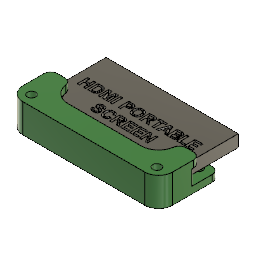
screen_holder (Autodesk Fusion 360 design; units mm, degrees)
Autodesk Fusion 360 part; units mm, degrees
sketch "Sketch1" plane through (0, 0, 0) normal (0, 0, 1) x (1, 0, 0) in component "screen"
  line L0 (95, 57.5) -> (-95, 57.5)
  line L1 (-95, 57.5) -> (-95, -57.5)
  line L2 (-95, -57.5) -> (95, -57.5)
  line L3 (95, -57.5) -> (95, 57.5)
  line L4 (95, 57.5) -> (-95, -57.5) construction
  line L5 (-95, 57.5) -> (95, -57.5) construction
  dimension "d1" = 190
  dimension "d2" = 115
  constraint horizontal L0
  constraint perpendicular L0 L1
  constraint parallel L0 L2
  constraint parallel L1 L3
  constraint coincident L4 origin
  constraint coincident L5 origin
  measures "d1" distance of L1.end L2.end
  measures "d2" distance of L0.end L1.end
extrude "Extrude1" add sketch "Sketch1" along normal blind 17.5 makes body 1 in component "screen"
sketch "Sketch2" plane through (0, 0, 17.5) normal (0, 0, 1) x (-1, 0, 0) in component "screen"
  line L0 (-95, 57.5) -> (-95, -57.5)
  line L1 (-95, -57.5) -> (95, -57.5)
  line L2 (95, -57.5) -> (95, 57.5)
  line L3 (95, 57.5) -> (-95, 57.5)
  line L4 (82.8095, -4.1103) -> (82.8095, -18.9885)
  line L5 (82.8095, -18.9885) -> (79.8055, -18.9885)
  line L6 (79.8055, -18.9885) -> (79.8055, -13.1326)
  line L7 (79.8055, -13.1326) -> (73.9191, -13.1326)
  line L8 (73.9191, -13.1326) -> (73.9191, -18.9885)
  line L9 (73.9191, -18.9885) -> (70.9151, -18.9885)
  line L10 (70.9151, -18.9885) -> (70.9151, -4.1103)
  line L11 (70.9151, -4.1103) -> (73.9191, -4.1103)
  line L12 (73.9191, -4.1103) -> (73.9191, -10.6157)
  line L13 (73.9191, -10.6157) -> (79.8055, -10.6157)
  line L14 (79.8055, -10.6157) -> (79.8055, -4.1103)
  line L15 (79.8055, -4.1103) -> (82.8095, -4.1103)
  line L16 (67.8095, -18.9885) -> (62.319, -18.9885)
  spline S0 degree 2 poles (62.319, -18.9885) (60.4618, -18.9885) (59.4875, -18.7043) knots 0 0 0 1 1 1
  spline S1 degree 2 poles (59.4875, -18.7043) (58.1783, -18.3187) (57.2446, -17.3342) knots 0 0 0 1 1 1
  spline S2 degree 2 poles (57.2446, -17.3342) (56.3109, -16.3498) (55.8237, -14.9239) knots 0 0 0 1 1 1
  spline S3 degree 2 poles (55.8237, -14.9239) (55.3366, -13.498) (55.3366, -11.4073) knots 0 0 0 1 1 1
  spline S4 degree 2 poles (55.3366, -11.4073) (55.3366, -9.5704) (55.7933, -8.2409) knots 0 0 0 1 1 1
  spline S5 degree 2 poles (55.7933, -8.2409) (56.3515, -6.617) (57.3867, -5.6123) knots 0 0 0 1 1 1
  spline S6 degree 2 poles (57.3867, -5.6123) (58.1681, -4.8511) (59.4976, -4.4249) knots 0 0 0 1 1 1
  spline S7 degree 2 poles (59.4976, -4.4249) (60.4922, -4.1103) (62.1566, -4.1103) knots 0 0 0 1 1 1
  line L17 (62.1566, -4.1103) -> (67.8095, -4.1103)
  line L18 (67.8095, -4.1103) -> (67.8095, -18.9885)
  line L19 (64.8055, -16.4716) -> (64.8055, -6.617)
  line L20 (64.8055, -6.617) -> (62.5626, -6.617)
  spline S8 degree 2 poles (62.5626, -6.617) (61.3041, -6.617) (60.7459, -6.7591) knots 0 0 0 1 1 1
  spline S9 degree 2 poles (60.7459, -6.7591) (60.0152, -6.9418) (59.5331, -7.3782) knots 0 0 0 1 1 1
  spline S10 degree 2 poles (59.5331, -7.3782) (59.0511, -7.8146) (58.7466, -8.8143) knots 0 0 0 1 1 1
  spline S11 degree 2 poles (58.7466, -8.8143) (58.4421, -9.8139) (58.4421, -11.5392) knots 0 0 0 1 1 1
  spline S12 degree 2 poles (58.4421, -11.5392) (58.4421, -13.2645) (58.7466, -14.1881) knots 0 0 0 1 1 1
  spline S13 degree 2 poles (58.7466, -14.1881) (59.0511, -15.1116) (59.5991, -15.6292) knots 0 0 0 1 1 1
  spline S14 degree 2 poles (59.5991, -15.6292) (60.1471, -16.1468) (60.9895, -16.3295) knots 0 0 0 1 1 1
  spline S15 degree 2 poles (60.9895, -16.3295) (61.6187, -16.4716) (63.4557, -16.4716) knots 0 0 0 1 1 1
  line L21 (63.4557, -16.4716) -> (64.8055, -16.4716)
  line L22 (52.8197, -4.1103) -> (52.8197, -18.9885)
  line L23 (52.8197, -18.9885) -> (48.3237, -18.9885)
  line L24 (48.3237, -18.9885) -> (45.6241, -8.8396)
  line L25 (45.6241, -8.8396) -> (42.955, -18.9885)
  line L26 (42.955, -18.9885) -> (38.4489, -18.9885)
  line L27 (38.4489, -18.9885) -> (38.4489, -4.1103)
  line L28 (38.4489, -4.1103) -> (41.2398, -4.1103)
  line L29 (41.2398, -4.1103) -> (41.2398, -15.822)
  line L30 (41.2398, -15.822) -> (44.1932, -4.1103)
  line L31 (44.1932, -4.1103) -> (47.0856, -4.1103)
  line L32 (47.0856, -4.1103) -> (50.0287, -15.822)
  line L33 (50.0287, -15.822) -> (50.0287, -4.1103)
  line L34 (50.0287, -4.1103) -> (52.8197, -4.1103)
  line L35 (35.5463, -4.1103) -> (35.5463, -18.9885)
  line L36 (35.5463, -18.9885) -> (32.5423, -18.9885)
  line L37 (32.5423, -18.9885) -> (32.5423, -4.1103)
  line L38 (32.5423, -4.1103) -> (35.5463, -4.1103)
  line L39 (23.8853, -4.1103) -> (23.8853, -18.9885)
  line L40 (23.8853, -18.9885) -> (19.0646, -18.9885)
  spline S16 degree 2 poles (19.0646, -18.9885) (16.3244, -18.9885) (15.4922, -18.7652) knots 0 0 0 1 1 1
  spline S17 degree 2 poles (15.4922, -18.7652) (14.2134, -18.4303) (13.3508, -17.3089) knots 0 0 0 1 1 1
  spline S18 degree 2 poles (13.3508, -17.3089) (12.4882, -16.1874) (12.4882, -14.4114) knots 0 0 0 1 1 1
  spline S19 degree 2 poles (12.4882, -14.4114) (12.4882, -13.0413) (12.9854, -12.1076) knots 0 0 0 1 1 1
  spline S20 degree 2 poles (12.9854, -12.1076) (13.4827, -11.1739) (14.249, -10.6411) knots 0 0 0 1 1 1
  spline S21 degree 2 poles (14.249, -10.6411) (15.0152, -10.1083) (15.8068, -9.9357) knots 0 0 0 1 1 1
  spline S22 degree 2 poles (15.8068, -9.9357) (16.8826, -9.7226) (18.9225, -9.7226) knots 0 0 0 1 1 1
  line L41 (18.9225, -9.7226) -> (20.8812, -9.7226)
  line L42 (20.8812, -9.7226) -> (20.8812, -4.1103)
  line L43 (20.8812, -4.1103) -> (23.8853, -4.1103)
  line L44 (20.8812, -16.4716) -> (20.8812, -12.2497)
  line L45 (20.8812, -12.2497) -> (19.2371, -12.2497)
  spline S23 degree 2 poles (19.2371, -12.2497) (17.4611, -12.2497) (16.8623, -12.4831) knots 0 0 0 1 1 1
  spline S24 degree 2 poles (16.8623, -12.4831) (16.2635, -12.7165) (15.9235, -13.2138) knots 0 0 0 1 1 1
  spline S25 degree 2 poles (15.9235, -13.2138) (15.5836, -13.7111) (15.5836, -14.3708) knots 0 0 0 1 1 1
  spline S26 degree 2 poles (15.5836, -14.3708) (15.5836, -15.1827) (16.0605, -15.7104) knots 0 0 0 1 1 1
  spline S27 degree 2 poles (16.0605, -15.7104) (16.5375, -16.2382) (17.2683, -16.3701) knots 0 0 0 1 1 1
  spline S28 degree 2 poles (17.2683, -16.3701) (17.8061, -16.4716) (19.43, -16.4716) knots 0 0 0 1 1 1
  line L46 (19.43, -16.4716) -> (20.8812, -16.4716)
  spline S29 degree 2 poles (10.6208, -11.458) (10.6208, -13.7314) (9.9408, -15.274) knots 0 0 0 1 1 1
  spline S30 degree 2 poles (9.9408, -15.274) (9.4333, -16.4107) (8.5555, -17.3139) knots 0 0 0 1 1 1
  spline S31 degree 2 poles (8.5555, -17.3139) (7.6776, -18.2172) (6.6323, -18.6536) knots 0 0 0 1 1 1
  spline S32 degree 2 poles (6.6323, -18.6536) (5.2419, -19.2422) (3.4252, -19.2422) knots 0 0 0 1 1 1
  spline S33 degree 2 poles (3.4252, -19.2422) (0.137, -19.2422) (-1.837, -17.2023) knots 0 0 0 1 1 1
  spline S34 degree 2 poles (-1.837, -17.2023) (-3.8109, -15.1624) (-3.8109, -11.5291) knots 0 0 0 1 1 1
  spline S35 degree 2 poles (-3.8109, -11.5291) (-3.8109, -7.9262) (-1.8522, -5.8914) knots 0 0 0 1 1 1
  spline S36 degree 2 poles (-1.8522, -5.8914) (0.1066, -3.8566) (3.3846, -3.8566) knots 0 0 0 1 1 1
  spline S37 degree 2 poles (3.3846, -3.8566) (6.7033, -3.8566) (8.662, -5.8813) knots 0 0 0 1 1 1
  spline S38 degree 2 poles (8.662, -5.8813) (10.6208, -7.906) (10.6208, -11.458) knots 0 0 0 1 1 1
  spline S39 degree 2 poles (7.5254, -11.5595) (7.5254, -9.0325) (6.3582, -7.7283) knots 0 0 0 1 1 1
  spline S40 degree 2 poles (6.3582, -7.7283) (5.1911, -6.4242) (3.3948, -6.4242) knots 0 0 0 1 1 1
  spline S41 degree 2 poles (3.3948, -6.4242) (1.5984, -6.4242) (0.4465, -7.7182) knots 0 0 0 1 1 1
  spline S42 degree 2 poles (0.4465, -7.7182) (-0.7053, -9.0122) (-0.7053, -11.6001) knots 0 0 0 1 1 1
  spline S43 degree 2 poles (-0.7053, -11.6001) (-0.7053, -14.1576) (0.4161, -15.4161) knots 0 0 0 1 1 1
  spline S44 degree 2 poles (0.4161, -15.4161) (1.5375, -16.6746) (3.3948, -16.6746) knots 0 0 0 1 1 1
  spline S45 degree 2 poles (3.3948, -16.6746) (5.252, -16.6746) (6.3887, -15.4009) knots 0 0 0 1 1 1
  spline S46 degree 2 poles (6.3887, -15.4009) (7.5254, -14.1272) (7.5254, -11.5595) knots 0 0 0 1 1 1
  line L47 (-6.1756, -4.1103) -> (-6.1756, -18.9885)
  line L48 (-6.1756, -18.9885) -> (-12.4983, -18.9885)
  spline S47 degree 2 poles (-12.4983, -18.9885) (-14.8833, -18.9885) (-15.9641, -18.5876) knots 0 0 0 1 1 1
  spline S48 degree 2 poles (-15.9641, -18.5876) (-17.045, -18.1867) (-17.6945, -17.1617) knots 0 0 0 1 1 1
  spline S49 degree 2 poles (-17.6945, -17.1617) (-18.3441, -16.1367) (-18.3441, -14.8173) knots 0 0 0 1 1 1
  spline S50 degree 2 poles (-18.3441, -14.8173) (-18.3441, -13.1428) (-17.3596, -12.0518) knots 0 0 0 1 1 1
  spline S51 degree 2 poles (-17.3596, -12.0518) (-16.3752, -10.9608) (-14.4164, -10.6766) knots 0 0 0 1 1 1
  spline S52 degree 2 poles (-14.4164, -10.6766) (-15.3907, -10.1083) (-16.025, -9.4283) knots 0 0 0 1 1 1
  spline S53 degree 2 poles (-16.025, -9.4283) (-16.6593, -8.7483) (-17.7351, -7.0128) knots 0 0 0 1 1 1
  line L49 (-17.7351, -7.0128) -> (-19.5518, -4.1103)
  line L50 (-19.5518, -4.1103) -> (-15.9591, -4.1103)
  line L51 (-15.9591, -4.1103) -> (-13.7872, -7.3478)
  spline S54 degree 2 poles (-13.7872, -7.3478) (-12.6303, -9.0832) (-12.204, -9.5348) knots 0 0 0 1 1 1
  spline S55 degree 2 poles (-12.204, -9.5348) (-11.7778, -9.9865) (-11.3008, -10.1539) knots 0 0 0 1 1 1
  spline S56 degree 2 poles (-11.3008, -10.1539) (-10.8238, -10.3214) (-9.7886, -10.3214) knots 0 0 0 1 1 1
  line L52 (-9.7886, -10.3214) -> (-9.1796, -10.3214)
  line L53 (-9.1796, -10.3214) -> (-9.1796, -4.1103)
  line L54 (-9.1796, -4.1103) -> (-6.1756, -4.1103)
  line L55 (-9.1796, -12.6962) -> (-11.4022, -12.6962)
  spline S57 degree 2 poles (-11.4022, -12.6962) (-13.5639, -12.6962) (-14.1018, -12.8789) knots 0 0 0 1 1 1
  spline S58 degree 2 poles (-14.1018, -12.8789) (-14.6397, -13.0616) (-14.9442, -13.5081) knots 0 0 0 1 1 1
  spline S59 degree 2 poles (-14.9442, -13.5081) (-15.2487, -13.9547) (-15.2487, -14.6245) knots 0 0 0 1 1 1
  spline S60 degree 2 poles (-15.2487, -14.6245) (-15.2487, -15.3755) (-14.8478, -15.8373) knots 0 0 0 1 1 1
  spline S61 degree 2 poles (-14.8478, -15.8373) (-14.4469, -16.299) (-13.7162, -16.4208) knots 0 0 0 1 1 1
  spline S62 degree 2 poles (-13.7162, -16.4208) (-13.3508, -16.4716) (-11.524, -16.4716) knots 0 0 0 1 1 1
  line L56 (-11.524, -16.4716) -> (-9.1796, -16.4716)
  line L57 (-9.1796, -16.4716) -> (-9.1796, -12.6962)
  line L58 (-24.1593, -4.1103) -> (-24.1593, -16.4716)
  line L59 (-24.1593, -16.4716) -> (-19.7446, -16.4716)
  line L60 (-19.7446, -16.4716) -> (-19.7446, -18.9885)
  line L61 (-19.7446, -18.9885) -> (-31.568, -18.9885)
  line L62 (-31.568, -18.9885) -> (-31.568, -16.4716)
  line L63 (-31.568, -16.4716) -> (-27.1634, -16.4716)
  line L64 (-27.1634, -16.4716) -> (-27.1634, -4.1103)
  line L65 (-27.1634, -4.1103) -> (-24.1593, -4.1103)
  line L66 (-45.3907, -4.1103) -> (-42.1228, -4.1103)
  line L67 (-42.1228, -4.1103) -> (-40.8238, -7.4898)
  line L68 (-40.8238, -7.4898) -> (-34.8765, -7.4898)
  line L69 (-34.8765, -7.4898) -> (-33.6485, -4.1103)
  line L70 (-33.6485, -4.1103) -> (-30.4618, -4.1103)
  line L71 (-30.4618, -4.1103) -> (-36.2568, -18.9885)
  line L72 (-36.2568, -18.9885) -> (-39.4334, -18.9885)
  line L73 (-39.4334, -18.9885) -> (-45.3907, -4.1103)
  line L74 (-39.8596, -9.9966) -> (-37.8095, -15.5176)
  line L75 (-37.8095, -15.5176) -> (-35.8001, -9.9966)
  line L76 (-35.8001, -9.9966) -> (-39.8596, -9.9966)
  line L77 (-45.8576, -18.9885) -> (-51.8048, -18.9885)
  spline S63 degree 2 poles (-51.8048, -18.9885) (-53.5707, -18.9885) (-54.4384, -18.8413) knots 0 0 0 1 1 1
  spline S64 degree 2 poles (-54.4384, -18.8413) (-55.3062, -18.6942) (-55.9912, -18.2273) knots 0 0 0 1 1 1
  spline S65 degree 2 poles (-55.9912, -18.2273) (-56.6763, -17.7605) (-57.133, -16.9841) knots 0 0 0 1 1 1
  spline S66 degree 2 poles (-57.133, -16.9841) (-57.5897, -16.2077) (-57.5897, -15.2436) knots 0 0 0 1 1 1
  spline S67 degree 2 poles (-57.5897, -15.2436) (-57.5897, -14.1982) (-57.0264, -13.3254) knots 0 0 0 1 1 1
  spline S68 degree 2 poles (-57.0264, -13.3254) (-56.4631, -12.4526) (-55.499, -12.0162) knots 0 0 0 1 1 1
  spline S69 degree 2 poles (-55.499, -12.0162) (-56.8589, -11.6204) (-57.5897, -10.6664) knots 0 0 0 1 1 1
  spline S70 degree 2 poles (-57.5897, -10.6664) (-58.3204, -9.7124) (-58.3204, -8.4235) knots 0 0 0 1 1 1
  spline S71 degree 2 poles (-58.3204, -8.4235) (-58.3204, -7.4087) (-57.8484, -6.4496) knots 0 0 0 1 1 1
  spline S72 degree 2 poles (-57.8484, -6.4496) (-57.3765, -5.4905) (-56.5595, -4.9171) knots 0 0 0 1 1 1
  spline S73 degree 2 poles (-56.5595, -4.9171) (-55.7426, -4.3437) (-54.545, -4.2118) knots 0 0 0 1 1 1
  spline S74 degree 2 poles (-54.545, -4.2118) (-53.794, -4.1306) (-50.9219, -4.1103) knots 0 0 0 1 1 1
  line L78 (-50.9219, -4.1103) -> (-45.8576, -4.1103)
  line L79 (-45.8576, -4.1103) -> (-45.8576, -18.9885)
  line L80 (-48.8616, -16.5122) -> (-48.8616, -13.0717)
  line L81 (-48.8616, -13.0717) -> (-50.8305, -13.0717)
  spline S75 degree 2 poles (-50.8305, -13.0717) (-52.5863, -13.0717) (-53.0125, -13.1225) knots 0 0 0 1 1 1
  spline S76 degree 2 poles (-53.0125, -13.1225) (-53.7838, -13.2138) (-54.2253, -13.6553) knots 0 0 0 1 1 1
  spline S77 degree 2 poles (-54.2253, -13.6553) (-54.6668, -14.0967) (-54.6668, -14.8173) knots 0 0 0 1 1 1
  spline S78 degree 2 poles (-54.6668, -14.8173) (-54.6668, -15.5074) (-54.2862, -15.9388) knots 0 0 0 1 1 1
  spline S79 degree 2 poles (-54.2862, -15.9388) (-53.9056, -16.3701) (-53.1546, -16.4614) knots 0 0 0 1 1 1
  spline S80 degree 2 poles (-53.1546, -16.4614) (-52.7081, -16.5122) (-50.587, -16.5122) knots 0 0 0 1 1 1
  line L82 (-50.587, -16.5122) -> (-48.8616, -16.5122)
  line L83 (-48.8616, -10.5954) -> (-48.8616, -6.617)
  line L84 (-48.8616, -6.617) -> (-51.6424, -6.617)
  spline S81 degree 2 poles (-51.6424, -6.617) (-53.2662, -6.617) (-53.7026, -6.7084) knots 0 0 0 1 1 1
  spline S82 degree 2 poles (-53.7026, -6.7084) (-54.3725, -6.8302) (-54.7936, -7.3021) knots 0 0 0 1 1 1
  spline S83 degree 2 poles (-54.7936, -7.3021) (-55.2148, -7.774) (-55.2148, -8.5656) knots 0 0 0 1 1 1
  spline S84 degree 2 poles (-55.2148, -8.5656) (-55.2148, -9.2354) (-54.8901, -9.7023) knots 0 0 0 1 1 1
  spline S85 degree 2 poles (-54.8901, -9.7023) (-54.5653, -10.1691) (-53.9513, -10.3823) knots 0 0 0 1 1 1
  spline S86 degree 2 poles (-53.9513, -10.3823) (-53.3373, -10.5954) (-51.2872, -10.5954) knots 0 0 0 1 1 1
  line L85 (-51.2872, -10.5954) -> (-48.8616, -10.5954)
  line L86 (-59.8021, -4.1103) -> (-59.8021, -18.8667)
  line L87 (-59.8021, -18.8667) -> (-62.8062, -18.8667)
  line L88 (-62.8062, -18.8667) -> (-62.8062, -6.617)
  line L89 (-62.8062, -6.617) -> (-70.2757, -6.617)
  line L90 (-70.2757, -6.617) -> (-70.2757, -4.1103)
  line L91 (-70.2757, -4.1103) -> (-59.8021, -4.1103)
  line L92 (-71.2906, -4.1103) -> (-71.2906, -18.9885)
  line L93 (-71.2906, -18.9885) -> (-82.3224, -18.9885)
  line L94 (-82.3224, -18.9885) -> (-82.3224, -16.4716)
  line L95 (-82.3224, -16.4716) -> (-74.2946, -16.4716)
  line L96 (-74.2946, -16.4716) -> (-74.2946, -13.1732)
  line L97 (-74.2946, -13.1732) -> (-81.7642, -13.1732)
  line L98 (-81.7642, -13.1732) -> (-81.7642, -10.6664)
  line L99 (-81.7642, -10.6664) -> (-74.2946, -10.6664)
  line L100 (-74.2946, -10.6664) -> (-74.2946, -6.617)
  line L101 (-74.2946, -6.617) -> (-82.6066, -6.617)
  line L102 (-82.6066, -6.617) -> (-82.6066, -4.1103)
  line L103 (-82.6066, -4.1103) -> (-71.2906, -4.1103)
  line L104 (42.9296, 14.2693) -> (40.0068, 13.9851)
  spline S87 degree 2 poles (40.0068, 13.9851) (39.7429, 15.4567) (38.9361, 16.1468) knots 0 0 0 1 1 1
  spline S88 degree 2 poles (38.9361, 16.1468) (38.1292, 16.8369) (36.7591, 16.8369) knots 0 0 0 1 1 1
  spline S89 degree 2 poles (36.7591, 16.8369) (35.3078, 16.8369) (34.5721, 16.2229) knots 0 0 0 1 1 1
  spline S90 degree 2 poles (34.5721, 16.2229) (33.8363, 15.6089) (33.8363, 14.7869) knots 0 0 0 1 1 1
  spline S91 degree 2 poles (33.8363, 14.7869) (33.8363, 14.2591) (34.1458, 13.8887) knots 0 0 0 1 1 1
  spline S92 degree 2 poles (34.1458, 13.8887) (34.4553, 13.5183) (35.2266, 13.2443) knots 0 0 0 1 1 1
  spline S93 degree 2 poles (35.2266, 13.2443) (35.7544, 13.0616) (37.6319, 12.5947) knots 0 0 0 1 1 1
  spline S94 degree 2 poles (37.6319, 12.5947) (40.0474, 11.9959) (41.0216, 11.1231) knots 0 0 0 1 1 1
  spline S95 degree 2 poles (41.0216, 11.1231) (42.3917, 9.8951) (42.3917, 8.1292) knots 0 0 0 1 1 1
  spline S96 degree 2 poles (42.3917, 8.1292) (42.3917, 6.9926) (41.7473, 6.0031) knots 0 0 0 1 1 1
  spline S97 degree 2 poles (41.7473, 6.0031) (41.1028, 5.0135) (39.89, 4.4959) knots 0 0 0 1 1 1
  spline S98 degree 2 poles (39.89, 4.4959) (38.6773, 3.9784) (36.9621, 3.9784) knots 0 0 0 1 1 1
  spline S99 degree 2 poles (36.9621, 3.9784) (34.161, 3.9784) (32.7453, 5.2064) knots 0 0 0 1 1 1
  spline S100 degree 2 poles (32.7453, 5.2064) (31.3295, 6.4344) (31.2585, 8.4844) knots 0 0 0 1 1 1
  line L105 (31.2585, 8.4844) -> (34.2625, 8.6164)
  spline S101 degree 2 poles (34.2625, 8.6164) (34.4553, 7.4696) (35.0896, 6.9672) knots 0 0 0 1 1 1
  spline S102 degree 2 poles (35.0896, 6.9672) (35.7239, 6.4648) (36.9925, 6.4648) knots 0 0 0 1 1 1
  spline S103 degree 2 poles (36.9925, 6.4648) (38.3018, 6.4648) (39.0426, 7.0027) knots 0 0 0 1 1 1
  spline S104 degree 2 poles (39.0426, 7.0027) (39.5196, 7.3478) (39.5196, 7.9263) knots 0 0 0 1 1 1
  spline S105 degree 2 poles (39.5196, 7.9263) (39.5196, 8.454) (39.0731, 8.8295) knots 0 0 0 1 1 1
  spline S106 degree 2 poles (39.0731, 8.8295) (38.5047, 9.3065) (36.3126, 9.8241) knots 0 0 0 1 1 1
  spline S107 degree 2 poles (36.3126, 9.8241) (34.1204, 10.3417) (33.07, 10.8948) knots 0 0 0 1 1 1
  spline S108 degree 2 poles (33.07, 10.8948) (32.0196, 11.4479) (31.4259, 12.407) knots 0 0 0 1 1 1
  spline S109 degree 2 poles (31.4259, 12.407) (30.8322, 13.366) (30.8322, 14.7767) knots 0 0 0 1 1 1
  spline S110 degree 2 poles (30.8322, 14.7767) (30.8322, 16.0555) (31.5426, 17.1719) knots 0 0 0 1 1 1
  spline S111 degree 2 poles (31.5426, 17.1719) (32.253, 18.2882) (33.5521, 18.8312) knots 0 0 0 1 1 1
  spline S112 degree 2 poles (33.5521, 18.8312) (34.8511, 19.3742) (36.7896, 19.3742) knots 0 0 0 1 1 1
  spline S113 degree 2 poles (36.7896, 19.3742) (39.611, 19.3742) (41.1231, 18.07) knots 0 0 0 1 1 1
  spline S114 degree 2 poles (41.1231, 18.07) (42.6353, 16.7659) (42.9296, 14.2693) knots 0 0 0 1 1 1
  line L106 (18.7754, 13.6401) -> (15.8626, 14.5636)
  spline S115 degree 2 poles (15.8626, 14.5636) (16.5325, 16.9993) (18.0903, 18.1817) knots 0 0 0 1 1 1
  spline S116 degree 2 poles (18.0903, 18.1817) (19.6482, 19.364) (22.0433, 19.364) knots 0 0 0 1 1 1
  spline S117 degree 2 poles (22.0433, 19.364) (25.0068, 19.364) (26.9147, 17.3393) knots 0 0 0 1 1 1
  spline S118 degree 2 poles (26.9147, 17.3393) (28.8227, 15.3146) (28.8227, 11.8031) knots 0 0 0 1 1 1
  spline S119 degree 2 poles (28.8227, 11.8031) (28.8227, 8.0886) (26.9046, 6.0335) knots 0 0 0 1 1 1
  spline S120 degree 2 poles (26.9046, 6.0335) (24.9865, 3.9784) (21.8606, 3.9784) knots 0 0 0 1 1 1
  spline S121 degree 2 poles (21.8606, 3.9784) (19.1306, 3.9784) (17.4256, 5.592) knots 0 0 0 1 1 1
  spline S122 degree 2 poles (17.4256, 5.592) (16.4107, 6.546) (15.9032, 8.3322) knots 0 0 0 1 1 1
  line L107 (15.9032, 8.3322) -> (18.8769, 9.0426)
  spline S123 degree 2 poles (18.8769, 9.0426) (19.1407, 7.8857) (19.978, 7.2158) knots 0 0 0 1 1 1
  spline S124 degree 2 poles (19.978, 7.2158) (20.8153, 6.546) (22.0129, 6.546) knots 0 0 0 1 1 1
  spline S125 degree 2 poles (22.0129, 6.546) (23.6671, 6.546) (24.6972, 7.7334) knots 0 0 0 1 1 1
  spline S126 degree 2 poles (24.6972, 7.7334) (25.7273, 8.9208) (25.7273, 11.5798) knots 0 0 0 1 1 1
  spline S127 degree 2 poles (25.7273, 11.5798) (25.7273, 14.4012) (24.7124, 15.5988) knots 0 0 0 1 1 1
  spline S128 degree 2 poles (24.7124, 15.5988) (23.6976, 16.7964) (22.0737, 16.7964) knots 0 0 0 1 1 1
  spline S129 degree 2 poles (22.0737, 16.7964) (20.8762, 16.7964) (20.0135, 16.0352) knots 0 0 0 1 1 1
  spline S130 degree 2 poles (20.0135, 16.0352) (19.1509, 15.274) (18.7754, 13.6401) knots 0 0 0 1 1 1
  line L108 (13.2645, 19.1103) -> (13.2645, 4.2321)
  line L109 (13.2645, 4.2321) -> (6.9418, 4.2321)
  spline S131 degree 2 poles (6.9418, 4.2321) (4.5568, 4.2321) (3.476, 4.633) knots 0 0 0 1 1 1
  spline S132 degree 2 poles (3.476, 4.633) (2.3951, 5.0338) (1.7456, 6.0589) knots 0 0 0 1 1 1
  spline S133 degree 2 poles (1.7456, 6.0589) (1.0961, 7.0839) (1.0961, 8.4033) knots 0 0 0 1 1 1
  spline S134 degree 2 poles (1.0961, 8.4033) (1.0961, 10.0778) (2.0805, 11.1688) knots 0 0 0 1 1 1
  spline S135 degree 2 poles (2.0805, 11.1688) (3.065, 12.2598) (5.0237, 12.544) knots 0 0 0 1 1 1
  spline S136 degree 2 poles (5.0237, 12.544) (4.0494, 13.1123) (3.4151, 13.7923) knots 0 0 0 1 1 1
  spline S137 degree 2 poles (3.4151, 13.7923) (2.7808, 14.4723) (1.705, 16.2077) knots 0 0 0 1 1 1
  line L110 (1.705, 16.2077) -> (-0.1116, 19.1103)
  line L111 (-0.1116, 19.1103) -> (3.4811, 19.1103)
  line L112 (3.4811, 19.1103) -> (5.6529, 15.8728)
  spline S138 degree 2 poles (5.6529, 15.8728) (6.8099, 14.1374) (7.2361, 13.6857) knots 0 0 0 1 1 1
  spline S139 degree 2 poles (7.2361, 13.6857) (7.6624, 13.2341) (8.1394, 13.0666) knots 0 0 0 1 1 1
  spline S140 degree 2 poles (8.1394, 13.0666) (8.6164, 12.8992) (9.6516, 12.8992) knots 0 0 0 1 1 1
  line L113 (9.6516, 12.8992) -> (10.2605, 12.8992)
  line L114 (10.2605, 12.8992) -> (10.2605, 19.1103)
  line L115 (10.2605, 19.1103) -> (13.2645, 19.1103)
  line L116 (10.2605, 10.5244) -> (8.0379, 10.5244)
  spline S141 degree 2 poles (8.0379, 10.5244) (5.8762, 10.5244) (5.3383, 10.3417) knots 0 0 0 1 1 1
  spline S142 degree 2 poles (5.3383, 10.3417) (4.8004, 10.159) (4.4959, 9.7125) knots 0 0 0 1 1 1
  spline S143 degree 2 poles (4.4959, 9.7125) (4.1915, 9.2659) (4.1915, 8.5961) knots 0 0 0 1 1 1
  spline S144 degree 2 poles (4.1915, 8.5961) (4.1915, 7.8451) (4.5923, 7.3833) knots 0 0 0 1 1 1
  spline S145 degree 2 poles (4.5923, 7.3833) (4.9932, 6.9215) (5.724, 6.7997) knots 0 0 0 1 1 1
  spline S146 degree 2 poles (5.724, 6.7997) (6.0893, 6.749) (7.9161, 6.749) knots 0 0 0 1 1 1
  line L117 (7.9161, 6.749) -> (10.2605, 6.749)
  line L118 (10.2605, 6.749) -> (10.2605, 10.5244)
  line L119 (-1.7456, 19.1103) -> (-1.7456, 4.2321)
  line L120 (-1.7456, 4.2321) -> (-12.7774, 4.2321)
  line L121 (-12.7774, 4.2321) -> (-12.7774, 6.749)
  line L122 (-12.7774, 6.749) -> (-4.7497, 6.749)
  line L123 (-4.7497, 6.749) -> (-4.7497, 10.0474)
  line L124 (-4.7497, 10.0474) -> (-12.2192, 10.0474)
  line L125 (-12.2192, 10.0474) -> (-12.2192, 12.5541)
  line L126 (-12.2192, 12.5541) -> (-4.7497, 12.5541)
  line L127 (-4.7497, 12.5541) -> (-4.7497, 16.6035)
  line L128 (-4.7497, 16.6035) -> (-13.0616, 16.6035)
  line L129 (-13.0616, 16.6035) -> (-13.0616, 19.1103)
  line L130 (-13.0616, 19.1103) -> (-1.7456, 19.1103)
  line L131 (-15.6191, 19.1103) -> (-15.6191, 4.2321)
  line L132 (-15.6191, 4.2321) -> (-26.6509, 4.2321)
  line L133 (-26.6509, 4.2321) -> (-26.6509, 6.749)
  line L134 (-26.6509, 6.749) -> (-18.6231, 6.749)
  line L135 (-18.6231, 6.749) -> (-18.6231, 10.0474)
  line L136 (-18.6231, 10.0474) -> (-26.0927, 10.0474)
  line L137 (-26.0927, 10.0474) -> (-26.0927, 12.5541)
  line L138 (-26.0927, 12.5541) -> (-18.6231, 12.5541)
  line L139 (-18.6231, 12.5541) -> (-18.6231, 16.6035)
  line L140 (-18.6231, 16.6035) -> (-26.935, 16.6035)
  line L141 (-26.935, 16.6035) -> (-26.935, 19.1103)
  line L142 (-26.935, 19.1103) -> (-15.6191, 19.1103)
  line L143 (-29.523, 19.1103) -> (-29.523, 4.2321)
  line L144 (-29.523, 4.2321) -> (-32.4459, 4.2321)
  line L145 (-32.4459, 4.2321) -> (-38.5352, 14.1678)
  line L146 (-38.5352, 14.1678) -> (-38.5352, 4.2321)
  line L147 (-38.5352, 4.2321) -> (-41.3261, 4.2321)
  line L148 (-41.3261, 4.2321) -> (-41.3261, 19.1103)
  line L149 (-41.3261, 19.1103) -> (-38.3119, 19.1103)
  line L150 (-38.3119, 19.1103) -> (-32.3139, 9.408)
  line L151 (-32.3139, 9.408) -> (-32.3139, 19.1103)
  line L152 (-32.3139, 19.1103) -> (-29.523, 19.1103)
extrude "Extrude2" cut sketch "Sketch2" against normal blind 5 contours L4 L5 L6 L7 L8 L9 L10 L11 L12 L13 L14 L15 | L16 S0 S1 S2 S3 S4 S5 S6 S7 L17 L18 | L22 L23 L24 L25 L26 L27 L28 L29 L30 L31 L32 L33 L34 | L35 L36 L37 L38 | L39 L40 S16 S17 S18 S19 S20 S21 S22 L41 L42 L43 | S29 S30 S31 S32 S33 S34 S35 S36 S37 S38 | L47 L48 S47 S48 S49 S50 S51 S52 S53 L49 L50 L51 S54 S55 S56 L52 L53 L54 | L58 L59 L60 L61 L62 L63 L64 L65 | L66 L67 L68 L69 L70 L71 L72 L73 | L77 S63 S64 S65 S66 S67 S68 S69 S70 S71 S72 S73 S74 L78 L79 | L86 L87 L88 L89 L90 L91 | L92 L93 L94 L95 L96 L97 L98 L99 L100 L101 L102 L103 | L104 S87 S88 S89 S90 S91 S92 S93 S94 S95 S96 S97 S98 S99 S100 L105 S101 S102 S103 S104 S105 S106 S107 S108 S109 S110 S111 S112 S113 S114 | L106 S115 S116 S117 S118 S119 S120 S121 S122 L107 S123 S124 S125 S126 S127 S128 S129 S130 | L108 L109 S131 S132 S133 S134 S135 S136 S137 L110 L111 L112 S138 S139 S140 L113 L114 L115 | L119 L120 L121 L122 L123 L124 L125 L126 L127 L128 L129 L130 | L131 L132 L133 L134 L135 L136 L137 L138 L139 L140 L141 L142 | L143 L144 L145 L146 L147 L148 L149 L150 L151 L152 bodies 1 in component "screen"
ref_plane "WorkPlane1" through (95, 0, 8.75) normal (1, 0, 0) x (0, 1, 0) in component "Screem_holder"
sketch "Sketch1 (2)" plane through (95, 0, 8.75) normal (1, 0, 0) x (0, 1, 0) in component "Screem_holder"
  line L0 (-57.5, -8.75) -> (57.5, -8.75)
  line L1 (57.5, -8.75) -> (57.5, 8.75)
  line L2 (57.5, 8.75) -> (-57.5, 8.75)
  line L3 (-57.5, 8.75) -> (-57.5, -8.75)
  line L4 (-9.5, 10.75) -> (-59.5, 10.75)
  line L5 (-59.5, 10.75) -> (-59.5, -10.75)
  line L6 (-59.5, -10.75) -> (17.5, -10.75)
  line L7 (-9.5, 10.75) -> (-9.5, 20.75)
  line L8 (-9.5, 20.75) -> (-69.5, 20.75)
  line L9 (-69.5, 20.75) -> (-69.5, -20.75)
  line L10 (-69.5, -20.75) -> (17.5, -20.75)
  line L11 (17.5, -20.75) -> (17.5, -10.75)
  dimension "d9" = 2
  dimension "d10" = 2
  dimension "d11" = 75
  dimension "d12" = 2
  dimension "d13" = 10
  dimension "d14" = 10
  dimension "d15" = 10
  dimension "d16" = 50
  constraint horizontal L4
  constraint perpendicular L4 L5
  constraint perpendicular L5 L6
  constraint perpendicular L4 L7
  constraint perpendicular L7 L8
  constraint perpendicular L8 L9
  constraint perpendicular L9 L10
  constraint perpendicular L10 L11
  measures "d9" distance of L2 L4
  measures "d10" distance of L0 L6
  measures "d11" distance of L3 L11
  measures "d12" distance of L3 L5
  measures "d13" distance of L6 L10
  measures "d14" distance of L4 L8
  measures "d15" distance of L5 L9
  measures "d16" distance of L5 L7
extrude "Extrude1'" add sketch "Sketch1 (2)" along normal blind 215 separate body contours L4 L5 L6 L7 L8 L9 L10 L11 makes body 2 in component "Screem_holder"
sketch "Sketch2 (2)" plane through (310, 0, 0) normal (1, 0, 0) x (0, 1, 0) in component "Screem_holder"
  line L0 (-9.5, 19.5) -> (-9.5, 29.5)
  line L1 (-9.5, 29.5) -> (-69.5, 29.5)
  line L2 (-69.5, 29.5) -> (-69.5, -12)
  line L3 (-69.5, -12) -> (17.5, -12)
  line L4 (17.5, -12) -> (17.5, -2)
  line L5 (17.5, -2) -> (-59.5, -2)
  line L6 (-59.5, -2) -> (-59.5, 19.5)
  line L7 (-59.5, 19.5) -> (-9.5, 19.5)
  line L8 (-19.5, 19.5) -> (-19.5, -2)
  line L9 (-19.5, 19.5) -> (-19.5, 29.5)
  line L10 (-19.5, -2) -> (-19.5, -12)
  dimension "d19" = 40
  constraint coincident L7 L8.start
  constraint coincident L5 L8.end
  constraint perpendicular L5 L8
  constraint coincident L1 L9.end
  constraint perpendicular L1 L9
  constraint coincident L3 L10.end
  constraint perpendicular L3 L10
  measures "d19" distance of L6 L8
extrude "Extrude2'" add sketch "Sketch2 (2)" against normal blind 10 contours L5 L6 L7 L8 | L1 L2 L3 L5 L6 L7 L9 L10 bodies 2 in component "Screem_holder"
extrude "Extrude3" add sketch "Sketch2 (2)" along normal blind 10 from surface at -215 contours L5 L6 L7 L8 | L1 L2 L3 L5 L6 L7 L9 L10 bodies 2 in component "Screem_holder"
sketch "Sketch3" plane through (0, 0, 29.5) normal (0, 0, 1) x (-1, 0, 0) in component "Screem_holder"
  line L0 (-95, 9.5) -> (-95, 69.5)
  line L1 (-95, 69.5) -> (-310, 69.5)
  line L2 (-310, 69.5) -> (-310, 9.5)
  line L3 (-310, 9.5) -> (-95, 9.5)
  line L4 (-202.5, 69.5) -> (-202.5, 9.5) construction
  line L5 (-125, -32.9447) -> (-280, -32.9447)
  line L6 (-280, -32.9447) -> (-280, 39.5)
  line L7 (-280, 39.5) -> (-125, 39.5)
  line L8 (-125, 39.5) -> (-125, -32.9447)
  line L9 (-105, 59.5) -> (-300, 59.5)
  dimension "d25" = 30
  dimension "d26" = 30
  dimension "d27" = 20
  constraint midpoint L1 L4.start
  constraint midpoint L3 L4.end
  constraint horizontal L5
  constraint vertical L6
  constraint horizontal L7
  constraint vertical L8
  measures "d25" distance of L2 L6
  measures "d26" distance of L0 L8
  measures "d27" distance of L7 L9
extrude "Extrude4" cut sketch "Sketch3" against normal blind 50 contours L3 L5 L6 L8 | L3 L6 L7 L8 bodies 2 in component "Screem_holder"
sketch "Sketch4" plane through (0, 0, 29.5) normal (0, 0, 1) x (-1, 0, 0) in component "Screem_holder"
  line L0 (-280, 9.5) -> (-280, 39.5)
  line L1 (-280, 39.5) -> (-125, 39.5)
  line L2 (-125, 39.5) -> (-125, 9.5)
  line L3 (-125, 9.5) -> (-95, 9.5)
  line L4 (-95, 9.5) -> (-95, 69.5)
  line L5 (-95, 69.5) -> (-310, 69.5)
  line L6 (-310, 69.5) -> (-310, 9.5)
  line L7 (-310, 9.5) -> (-280, 9.5)
  circle A0 centre (-112.5, -5.5) radius 2.25
  circle A1 centre (-292.5, -5.5) radius 2.25
  circle A2 centre (-112.5, 54.5) radius 2.25
  circle A3 centre (-292.5, 54.5) radius 1.75
  line L8 (-202.5, 69.5) -> (-202.5, 39.5) construction
  dimension "d30" = 4.5
  dimension "d31" = 4.5
  dimension "d32" = 4.5
  dimension "d33" = 3.5
  dimension "d34" = 60
  dimension "d35" = 180
  dimension "d36" = 90
  dimension "d37" = 15
  constraint vertical A0.centre A2.centre
  constraint horizontal A2.centre A3.centre
  constraint vertical A1.centre A3.centre
  constraint horizontal A0.centre A1.centre
  constraint midpoint L5 L8.start
  constraint midpoint L1 L8.end
  measures "d30" diameter of A0
  measures "d31" diameter of A1
  measures "d32" diameter of A2
  measures "d33" diameter of A3
  measures "d34" distance of A0.centre A2.centre
  measures "d35" distance of A0.centre A1.centre
  measures "d36" distance of A2.centre L8
  measures "d37" distance of L5 A3.centre
extrude "Extrude5" cut sketch "Sketch4" against normal blind 50 contours A0 | A1 | A2 | A3 bodies 2 in component "Screem_holder"
sketch "Sketch5" plane through (0, 0, 29.5) normal (0, 0, 1) x (-1, 0, 0) in component "Screem_holder"
  circle A0 centre (-112.5, 54.5) radius 2.25
  circle A1 centre (-292.5, 54.5) radius 1.75
  line L0 (-280, 9.5) -> (-280, 39.5)
  line L1 (-280, 39.5) -> (-125, 39.5)
  line L2 (-125, 39.5) -> (-125, 9.5)
  line L3 (-125, 9.5) -> (-95, 9.5)
  line L4 (-95, 9.5) -> (-95, 69.5)
  line L5 (-95, 69.5) -> (-310, 69.5)
  line L6 (-310, 69.5) -> (-310, 9.5)
  line L7 (-310, 9.5) -> (-280, 9.5)
  circle A2 centre (-112.5, 54.5) radius 6
  circle A3 centre (-292.5, 54.5) radius 6
  dimension "d40" = 12
  dimension "d41" = 12
  constraint concentric A0 A2
  constraint concentric A1 A3
  measures "d40" diameter of A2
  measures "d41" diameter of A3
extrude "Extrude6" cut sketch "Sketch5" against normal up to surface (31.5 mm away) contours A2 | A3 bodies 2 in component "Screem_holder"
sketch "Sketch6" plane through (0, 0, -2) normal (0, 0, 1) x (-1, 0, 0) in component "Screem_holder"
  circle A0 centre (-112.5, 54.5) radius 2.25
  circle A1 centre (-292.5, 54.5) radius 1.75
  line L0 (-115.8166, 59.5) -> (-289.1834, 59.5)
  arc A2 (-289.1834, 59.5) -> (-295.8166, 59.5) centre (-292.5, 54.5) ccw
  line L1 (-295.8166, 59.5) -> (-300, 59.5)
  line L2 (-300, 59.5) -> (-300, 19.5)
  line L3 (-300, 19.5) -> (-310, 19.5)
  line L4 (-310, 19.5) -> (-310, -17.5)
  line L5 (-310, -17.5) -> (-280, -17.5)
  line L6 (-280, -17.5) -> (-280, 39.5)
  line L7 (-280, 39.5) -> (-125, 39.5)
  line L8 (-125, 39.5) -> (-125, -17.5)
  line L9 (-125, -17.5) -> (-95, -17.5)
  line L10 (-95, -17.5) -> (-95, 19.5)
  line L11 (-95, 19.5) -> (-105, 19.5)
  line L12 (-105, 19.5) -> (-105, 59.5)
  line L13 (-105, 59.5) -> (-109.1834, 59.5)
  arc A3 (-109.1834, 59.5) -> (-115.8166, 59.5) centre (-112.5, 54.5) ccw
  circle A4 centre (-112.5, -5.5) radius 2.25
  circle A5 centre (-292.5, -5.5) radius 2.25
  circle A6 centre (-112.5, -5.5) radius 6
  circle A7 centre (-112.5, 54.5) radius 6
  circle A8 centre (-292.5, -5.5) radius 6
  circle A9 centre (-292.5, 54.5) radius 6
  dimension "d44" = 12
  dimension "d45" = 12
  dimension "d46" = 12
  dimension "d47" = 12
  constraint concentric A4 A6
  constraint concentric A0 A7
  constraint concentric A5 A8
  constraint concentric A1 A9
  measures "d44" diameter of A6
  measures "d45" diameter of A7
  measures "d46" diameter of A8
  measures "d47" diameter of A9
extrude "Extrude7" cut sketch "Sketch6" against normal blind 6 contours A3 A7 | A2 A9 | A6 | A8 bodies 2 in component "Screem_holder"
fillet "Fillet1" radius 25 4 edges at (125, -39.5, -7) (125, -39.5, 24.5) (280, -39.5, -7) (280, -39.5, 24.5) on bodies 2 in component "Screem_holder"
fillet "Fillet1" radius 10 8 edges at (125, -9.5, 24.5) (95, -9.5, 24.5) (95, 17.5, -7) (125, 17.5, -7) (280, 17.5, -7) (310, 17.5, -7) (280, -9.5, 24.5) (310, -9.5, 24.5) on bodies 2 in component "Screem_holder"
fillet "Fillet1" radius 2.5 4 edges at (300, -19.5, 8.75) (310, -19.5, 8.75) (95, -19.5, 8.75) (105, -19.5, 8.75) on bodies 2 in component "Screem_holder"
fillet "Fillet1" radius 20 2 edges at (310, -69.5, 8.75) (95, -69.5, 8.75) on bodies 2 in component "Screem_holder"
component "screen" placed x (1, 0, 0) y (0, 1, 0) z (0, 0, 1) at (202.5, 0, 0)
component "Screem_holder" placed x (1, 0, 0) y (0, 1, 0) z (0, 0, 1) at (0, 0, 0)
equation "d10 = d9"
equation "d12 = d9"
equation "d14 = d13"
equation "d15 = d13"
equation "d34 = ( 15 * 4 ) * 1 mm"
equation "d35 = ( 15 * 12 ) * 1 mm"
equation "d36 = d35 / 2"
